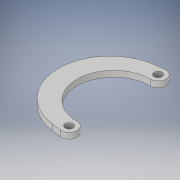
# Autodesk Inventor part: 000.703 - Тяга
Saved by Autodesk Inventor 2019 (Build 230136000, 136)
## iProperties
Created: 2020-02-29
Part Number: 000.703 - Тяга
Material: Типовые
Document SubType Name: Modeling
Designer: Петров Иван
Density: 1 g/cm^3
Appearance: По умолчанию
Author: Петров Иван
Autodesk Inventor part; units mm, degrees
ref_plane "YZ Plane" through (0, 0, 0) normal (1, 0, 0) x (0, 1, 0)
ref_plane "XZ Plane" through (0, 0, 0) normal (0, 1, 0) x (-1, 0, 0)
ref_plane "XY Plane" through (0, 0, 0) normal (0, 0, 1) x (1, 0, 0)
sketch "Эскиз3" plane through (0, 0, 0) normal (0, 1, 0) x (-1, 0, 0)
  arc A0 (1.791, 3.5766) -> (0, -4) centre (0, 0) ccw
  arc A1 (0, -41) -> (1.791, -48.5766) centre (0, -45) ccw
  arc A2 (1.791, -48.5766) -> (1.791, 3.5766) centre (1.791, -22.5) ccw
  arc A3 (0, -41) -> (0, -4) centre (0, -22.5) ccw
  dimension "d12" = 8
  dimension "d13" = 8
  dimension "d14" = 45
  constraints: 12 point on circle, 4 centre point, 1 coincident
  measures "d12" diameter of A0
  measures "d13" diameter of A1
  measures "d14" distance of point (0, 0) A1.centre
extrude "Выдавливание3" add sketch "Эскиз3" along normal blind 3
sketch "Эскиз4" plane through (0, 3, 0) normal (0, 1, 0) x (1, 0, 0)
  circle A0 centre (0, 0) radius 2
  arc A1 (0, 41) -> (-1.791, 48.5766) centre (0, 45) ccw projected
  circle A2 centre (0, 45) radius 2
  dimension "d17" = 4
  dimension "d18" = 4
  constraints: 2 centre point, 2 coincident
  measures "d17" diameter of A0
  measures "d18" diameter of A2
extrude "Выдавливание4" cut sketch "Эскиз4" against normal blind 9.25
fillet "Сопряжение1" radius 364.75 2 edges at (-1.791, 1.5, 3.5766) (-1.791, 1.5, -48.5766)
